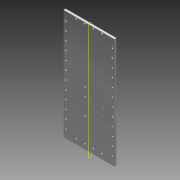
# Autodesk Inventor part: YagiBottom
Saved by Autodesk Inventor 2014 (Build 180170000, 170)
## iProperties
Created: 2015-05-19
Part Number: YagiBottom
Material: Generic
Document SubType Name: Modeling
Designer: Owner
Density: 1 g/cm^3
Appearance: Aluminum - Polished
Author: Owner
Autodesk Inventor part; units mm, degrees
ref_plane "YZ Plane" through (0, 0, 0) normal (1, 0, 0) x (0, 1, 0)
ref_plane "XZ Plane" through (0, 0, 0) normal (0, 1, 0) x (-1, 0, 0)
ref_plane "XY Plane" through (0, 0, 0) normal (0, 0, 1) x (1, 0, 0)
sketch "Sketch1" plane through (0, 0, 0) normal (0, 0, 1) x (1, 0, 0)
  line L0 (0, 158.602) -> (76.2, 158.602)
  line L1 (76.2, 158.602) -> (76.2, -6.498)
  line L2 (76.2, -6.498) -> (0, -6.498)
  line L3 (0, -6.498) -> (0, 158.602)
  point P0 (0, 0)
  dimension "d0" = 76.2
  dimension "d1" = 165.1
  constraints: 8 end point, 2 parallel, 1 horizontal, 1 perpendicular
  measures "d0" distance of L0.start L0.end
  measures "d1" distance of L0.end L1.end
extrude "Extrusion1" add sketch "Sketch1" along normal blind 3.175
sketch "Sketch2" plane through (0, 0, 3.175) normal (0, 0, 1) x (1, 0, 0)
  point P0 (19.05, -3.323)
hole "Hole1" at (19.05, -3.323, 3.175) direction (0, 0, -1) diameter 1.778 depth 3.175 countersink diameter 3.0226 countersink angle 82
sketch "Sketch3" plane through (0, 0, 3.175) normal (0, 0, 1) x (1, 0, 0)
  point P0 (19.05, 155.427)
hole "Hole3" at (19.05, 155.427, 3.175) direction (0, 0, -1) diameter 1.778 depth 3.175 countersink diameter 3.0226 countersink angle 82
sketch "Sketch4" plane through (0, 0, 3.175) normal (0, 0, 1) x (1, 0, 0)
  point P0 (73.025, 6.202)
hole "Hole5" at (73.025, 6.202, 3.175) direction (0, 0, -1) diameter 1.778 depth 3.175 countersink diameter 3.0226 countersink angle 82
pattern_linear "Rectangular Pattern1" count 12 spacing 12.7 along (0, 1, 0) of "Hole5"
pattern_linear "Rectangular Pattern2" count 2 spacing 12.7 along (1, 0, 0) of "Hole1"
pattern_linear "Rectangular Pattern3" count 2 spacing 12.7 along (1, 0, 0) of "Hole3"
ref_plane "Work Plane1" through (38.1, -6.498, 0) normal (1, 0, 0) x (0, 0, -1)
mirror "Mirror1" about plane through (38.1, -6.498, 0) normal (1, 0, 0) of "Hole3", "Rectangular Pattern3", "Hole5", "Rectangular Pattern1", "Hole1", "Rectangular Pattern2"
sketch "Sketch5" plane through (0, 0, 3.175) normal (0, 0, 1) x (1, 0, 0)
  point P0 (31.75, 62.802)
hole "Hole7" at (31.75, 62.802, 3.175) direction (0, 0, -1) diameter 1.778 depth 3.175 countersink diameter 3.0226 countersink angle 82
pattern_linear "Rectangular Pattern4" count 2 spacing 25.4 along (0, -1, 0) of "Hole7"
pattern_linear "Rectangular Pattern5" count 2 spacing 12.7 along (0, 1, 0) of "Hole7"
sketch "Sketch6" plane through (0, 0, 3.175) normal (0, 0, 1) x (1, 0, 0)
  point P0 (58.8, 62.083)
hole "Hole9" at (58.8, 62.083, 3.175) direction (0, 0, -1) diameter 1.778 depth 3.175
sketch "Sketch7" plane through (0, 0, 3.175) normal (0, 0, 1) x (1, 0, 0)
  point P0 (58.8, 50.018)
hole "Hole11" at (58.8, 50.018, 3.175) direction (0, 0, -1) diameter 1.778 depth 3.175
sketch "Sketch8" plane through (0, 0, 3.175) normal (0, 0, 1) x (1, 0, 0)
  point P0 (39.75, 62.083)
hole "Hole13" at (39.75, 62.083, 3.175) direction (0, 0, -1) diameter 1.778 depth 3.175
body "Solid1"
